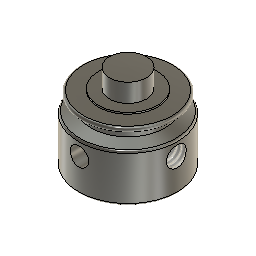
CutterHead_FR188ZZ (Autodesk Fusion 360 design; units mm, degrees)
Autodesk Fusion 360 part; units mm, degrees
sketch "Sketch1" plane through (0, 0, 0) normal (0, 1, 0) x (1, 0, 0) in component "Head"
  line L0 (0, 9.0932) -> (3.175, 9.0932)
  line L1 (3.175, 9.0932) -> (3.175, 5.9182)
  line L2 (5.08, 5.9182) -> (3.175, 5.9182)
  line L3 (5.08, 5.6642) -> (5.08, 5.9182)
  line L4 (5.08, 5.6642) -> (8.4938, 5.6642)
  line L5 (8.4938, 5.6642) -> (8.4938, -2.4755)
  line L6 (6.3514, -3.1716) -> (8.4938, -2.4755)
  circle A0 centre (7.6214, -3.8104) radius 1 construction
  line L7 (6.3514, -3.1716) -> (6.3514, -4.4492)
  line L8 (7.7385, -4.8999) -> (6.3514, -4.4492)
  arc A1 (7.6208, -5.6482) -> (7.7385, -4.8999) centre (7.62, -5.2647) ccw
  line L9 (5.08, -5.6536) -> (7.6208, -5.6482)
  line L10 (5.08, -5.6536) -> (5.08, -5.9076)
  line L11 (5.08, -5.9076) -> (3.175, -5.9076)
  line L12 (3.175, -9.0826) -> (3.175, -5.9076)
  line L13 (0, -9.0932) -> (3.175, -9.0826)
  circle A2 centre (0, 0) radius 1.5875
  line L14 (0, -9.0932) -> (0, 9.0932)
  circle A3 centre (0, 0) radius 1.8288
  circle A4 centre (0, 0) radius 2.159 construction
  dimension "d5" = 3.6576
  dimension "d6" = 4.318
  dimension "d7" = 3.175
  dimension "d10" = 3.175
  dimension "d12" = 0.254
  dimension "d15" = 3.175
  dimension "d16" = 0.3835
  dimension "d17" = 1.905
  dimension "d19" = 1.905
  dimension "d20" = 3.175
  dimension "d21" = 3.175
  dimension "d22" = 0.254
  dimension "d23" = 3.4138
  dimension "d24" = 1.2776
  dimension "d25" = 108
  dimension "d26" = 108
  dimension "d27" = 6.3514
  dimension "d28" = 3.1716
  dimension "d29" = 7.62
  dimension "d30" = 7.6214
  dimension "d38" = 5.6642
  dimension "d39" = 5.6642
  constraint coincident A2.centre A3.centre
  constraint vertical L14
  constraint midpoint A2.centre L14
  constraint vertical L12
  constraint coincident L12.start L13.end
  constraint coincident L10.end L11.start
  constraint coincident L11.end L12.end
  constraint tangent L8 A1
  constraint coincident L8 A1.end
  constraint coincident L8.start A1
  constraint coincident A1.start L9
  constraint coincident A1 L9.end
  constraint tangent A1 L9
  constraint vertical L10
  constraint horizontal L11
  constraint coincident L0 L14.end
  constraint coincident L0.start L14
  constraint coincident L0.end L1.start
  constraint coincident L2.start L3
  constraint coincident L2 L3.end
  constraint coincident L3 L4.start
  constraint coincident L3.start L4
  constraint coincident L4 L5.start
  constraint coincident L4.end L5
  constraint horizontal L0
  constraint vertical L1
  constraint horizontal L2
  constraint vertical L3
  constraint horizontal L4
  constraint coincident L5 L6.end
  constraint coincident L5.end L6
  constraint coincident L6 L7.start
  constraint coincident L6.start L7
  constraint coincident L7.end L8
  constraint coincident L7 L8.end
  constraint vertical L5
  constraint vertical L7
  constraint tangent L6 A0
  constraint tangent A0 L8
  measures "d5" diameter of A3
  measures "d6" diameter of A4
  measures "d7" diameter of A2
  measures "d10" distance of L0.start L0.end
  measures "d12" vertical distance of L9.start L10.end
  measures "d15" distance of L12.start L13.start
  measures "d16" radius of A1
  measures "d17" distance of L10.end L11.end
  measures "d19" distance of L1.end L2.start
  measures "d20" distance of L12.start L11.end
  measures "d21" distance of L0.end L1.end
  measures "d22" vertical distance of L3.start L2.start
  measures "d23" distance of L3.start L4.end
  measures "d24" distance of L6.start L7.end
  measures "d25" angle of L6 L7
  measures "d26" angle of L7 L8
  measures "d27" distance of L7 A2.centre
  measures "d28" vertical distance of L6.start A2.centre
  measures "d29" horizontal distance of A2.centre A1.centre
  measures "d30" horizontal distance of A2.centre A0.centre
  measures "d38" distance of L9 A2.centre
  measures "d39" distance of A2.centre L4
revolve "Revolve1" add sketch "Sketch1" angle 360 about axis through (0, 0, 9.0932) along (0, 0, -1) contours L0 L1 L2 L3 L4 L5 L6 L7 L8 A1 L9 L10 L11 L12 L13 L14 A3 | A2 L14 A3 | A2 L14 picked at (0.1621, 1.7368) picked at (0.4752, 0.3411) in component "Head"
extrude "Extrude1" cut sketch "Sketch1" along normal mid plane 24.8056 contours A2 L14 A3 | A2 L14 A3 | A2 L14 | A2 L14 in component "Head"
thread "Thread1" "ANSI Unified Screw Threads 0.164(#8) 8-32 UNC 3B" major diameter 4.1656 minor diameter 3.4163 pitch 0.7937 angle 60 resizes the face on face at (0.6666, 2.8176, -1.703) in component "Head"
move_face "MoveFace1" to x (0, 1, 0) y (-1, 0, 0) z (0, 0, 1) at (0, 0, 0) 1 faces at (0.3984, -2.8251, -1.661) in component "Head"
extrude "Extrude2" cut sketch "Sketch1" along normal mid plane 23.7185 contours A2 L14 | A2 L14 in component "Head"
fillet "Fillet1" radius 0.381 2 edges at (-7.919, -3.0715, -5.6642) (-7.919, -3.0715, 2.4755) in component "Head"
component "Head" placed x (1, 0, 0) y (0, 1, 0) z (0, 0, 1) at (0, 0, 0)
equation "d19 = d17"
equation "d21 = d20"
equation "d22 = d12"
